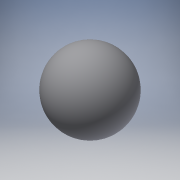
# Autodesk Inventor part: Ball
Saved by Autodesk Inventor 2019 (Build 230136000, 136)
## iProperties
Created: 2019-07-11
Part Number: Ball
Material: Generic
Document SubType Name: Modeling
Designer: AlphaGoldOmegaSilver
Mass: 134.066 g
Surface Area: 126.677 cm^2
Volume: 134.066 cm^3
Density: 1 g/cm^3
Appearance: Default
Author: AlphaGoldOmegaSilver
Autodesk Inventor part; units mm, degrees
ref_plane "YZ Plane" through (0, 0, 0) normal (1, 0, 0) x (0, 1, 0)
ref_plane "XZ Plane" through (0, 0, 0) normal (0, 1, 0) x (-1, 0, 0)
ref_plane "XY Plane" through (0, 0, 0) normal (0, 0, 1) x (1, 0, 0)
sketch "Sketch1" plane through (0, 0, 0) normal (1, 0, 0) x (0, 1, 0)
  line L0 (0, 0) -> (-9.6807, -62.7577)
  arc A0 (-9.6807, -62.7577) -> (0, 0) centre (-4.8404, -31.3789) ccw
  dimension "d0" = 63.5
  dimension "d1" = 31.75
  constraints: 2 end point, 2 point on circle, 1 centre point
  measures "d0" distance of L0.start L0.end
  measures "d1" radius of A0
revolve "Revolution1" add sketch "Sketch1" angle 360 about axis through (0, 0, 0) along (0, -0.1524522, -0.9883108)
body "Solid1"
